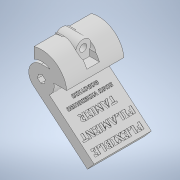
# Autodesk Inventor part: switch curvey lever boi
Saved by Autodesk Inventor 2022 (Build 260153000, 153)
## iProperties
Created: 2022-10-11
Part Number: switch curvey lever boi
Material: Generic
Document SubType Name: Modeling
Designer: Admin
Density: 1 g/cm^3
Appearance: Default
Author: Admin
Autodesk Inventor part; units mm, degrees
ref_plane "YZ Plane" through (0, 0, 0) normal (1, 0, 0) x (0, 1, 0)
ref_plane "XZ Plane" through (0, 0, 0) normal (0, 1, 0) x (-1, 0, 0)
sketch "Sketch1" plane through (0, 0, 0) normal (0, 0, 1) x (1, 0, 0)
  arc A0 (17.7715, 26.4992) -> (-7.9449, 43.6347) centre (-2.1282, 24.4992) ccw
  arc A1 (4.505, 34.4992) -> (-7.9449, 34.9952) centre (-2.1282, 24.4992) ccw
  line L0 (-2.1282, 34.4992) -> (4.505, 34.4992)
  line L1 (7.6697, 26.4992) -> (17.7715, 26.4992)
  line L2 (-8.5561, 16.8387) -> (34.0976, -18.9519)
  line L3 (34.0976, -18.9519) -> (39.2399, -12.8236)
  line L4 (39.2399, -12.8236) -> (4.0919, 16.6691)
  circle A2 centre (-2.1282, 24.4992) radius 4.5861 construction
  line L5 (-4.6095, 26.4808) -> (-1.6527, 27.6388)
  line L6 (-1.6527, 27.6388) -> (0.8285, 25.6572)
  line L7 (0.8285, 25.6572) -> (0.353, 22.5176)
  line L8 (0.353, 22.5176) -> (-2.6038, 21.3596)
  line L9 (-2.6038, 21.3596) -> (-5.085, 23.3412)
  line L10 (-5.085, 23.3412) -> (-4.6095, 26.4808)
  arc A3 (-2.1282, 34.4992) -> (-8.5561, 16.8387) centre (-2.1282, 24.4992) ccw
  arc A4 (4.0919, 16.6691) -> (7.6697, 26.4992) centre (-2.1282, 24.4992) ccw
  circle A5 centre (-2.1282, 24.4992) radius 20.0723 construction
  line L11 (-7.9449, 34.9952) -> (-7.9449, 43.7102)
  line L12 (8.708, 44.4992) -> (-7.9449, 44.4992)
  line L13 (-7.9449, 44.4992) -> (-7.9449, 31.8089)
  line L14 (-7.9449, 31.8089) -> (8.708, 31.8089)
  line L15 (8.708, 31.8089) -> (8.708, 44.4992)
  line L16 (8.708, 31.8089) -> (23.6844, 31.8089)
  line L17 (23.6844, 31.8089) -> (23.6844, 44.6206)
  line L18 (23.6844, 44.6206) -> (8.708, 44.6206)
  line L19 (8.708, 44.6206) -> (8.708, 31.8089)
  point P0 (0, 0)
  point P1 (-4.0178, 44.4097)
  point P2 (11.1125, 52.4992)
  point P3 (10.8839, 39.6875)
  point P4 (-7.9449, 34.9952)
  point P5 (8.708, 41.3092)
  point P6 (-7.9449, 32.6335)
  point P7 (-2.1282, 44.4992)
  dimension "d9" = 8
  dimension "d10" = 9.1722
  dimension "d11" = 5.5
  dimension "d12" = 40
  dimension "d13" = 8
  dimension "d16" = 8
  dimension "d17" = 10
  dimension "d18" = 20
  constraints: 40 end point, 9 point on circle, 6 parallel, 5 centre point, 4 coincident, 4 tangent, 3 perpendicular, 2 horizontal, 2 point on line, 1 vertical, 16 other
  measures "d9" distance between parallel lines of L1 L0
  measures "d10" diameter of A2
  measures "d11" distance between parallel lines of L8 L5
  measures "d12" angle of L2 L0
  measures "d13" distance between parallel lines of L2 L4
  measures "d16" radial gap between concentric circles of A0 A1
  measures "d17" radius of A3
  measures "d18" radius of A0
extrude "Extrusion1" add sketch "Sketch1" against normal blind 45 contours L1 A4 L4 L3 L2 A3 L13 L14 L16 A0 | L16 L15 A0 | L15 L14 L13 A3 L0 A1 L11 A0
ref_plane "Work Plane1" through (0, 0, -27) normal (0, 0, -1) x (-1, 0, 0)
extrude "Extrusion4" add sketch "Sketch1" along normal blind 10 from surface at -27 contours L15 L14 L13 A3 L0 A1 L11 A0 | A0 L12 L15 | A0 L11 L13 L12 | L13 A1 L0 A3
extrude "Extrusion5" cut sketch "Sketch1" along normal blind 10 from surface at -27 contours L16 L15 A0 | A0 L15 L19 L18 L17 L16 | L13 A1 L0 A3
sketch "Sketch2" plane through (8.708, 44.4992, -17) normal (1, 0, 0) x (0, 0, -1)
  circle A0 centre (5, -4.5078) radius 2.8
  line L0 (10, 0) -> (0, 0) projected
  line L1 (0, -12.6903) -> (0, -3.19) projected
  line L2 (10, 0) -> (0, 0) construction
  line L3 (5, 0) -> (5, -12.8117) construction
  circle A1 centre (5, -4.5078) radius 6
  line L4 (0, -3.19) -> (0, 0) projected
  line L5 (10, -3.19) -> (10, 0) projected
  point P0 (-17, -44.4992)
  point P1 (1.0402, 0)
  point P2 (8.9598, 0)
  point P3 (10, -1.1911)
  point P4 (0, -1.1911)
  dimension "d24" = 5.6
  dimension "d25" = 4.5078
  dimension "d29" = 12
  constraints: 2 centre point, 2 end point, 1 midpoint, 1 perpendicular, 1 point on line
  measures "d24" diameter of A0
  measures "d25" distance from line of A0.centre L0
  measures "d29" diameter of A1
extrude "Extrusion6" cut sketch "Sketch2" against normal through all contours A0
extrude "Extrusion7" cut sketch "Sketch2" along normal blind 10 contours A1 L1 L4 L0 | L0 A1 | L4 L1 A1
extrude "Extrusion8" add sketch "Sketch2" against normal up to surface (16.6529 mm away) contours A1 L1 L4 L0 | L0 A1 | L4 L1 A1
extrude "Extrusion9" cut sketch "Sketch2" against normal up to surface contours L5 A1 L0 | A1 L4 L0 round surface about axis through (-2.1282, 24.4992, 0) along (0, 0, -1) radius 20 far side no
sketch "Sketch3" plane through (39.2399, -12.8236, 0) normal (0.6427876, 0.7660444, 0) x (0.7660444, -0.6427876, 0)
  line L0 (-3.0027, 42.1524) -> (-3.0027, 2.7889) construction
  line L1 (-3.0027, 2.7889) -> (-46.5097, 2.7889) construction
  line L2 (-46.5097, 2.7889) -> (-46.5097, 42.1524) construction
  line L3 (-46.5097, 42.1524) -> (-3.0027, 42.1524) construction
  line L4 (-3.0027, 41.6774) -> (-3.0027, 40.0154)
  line L5 (-3.0027, 40.0154) -> (-5.2343, 40.0154)
  line L6 (-5.2343, 40.0154) -> (-5.2343, 38.4806)
  line L7 (-5.2343, 38.4806) -> (-6.2183, 38.4806)
  line L8 (-6.2183, 38.4806) -> (-6.2183, 40.0154)
  line L9 (-6.2183, 40.0154) -> (-8.0027, 40.0154)
  line L10 (-8.0027, 40.0154) -> (-8.0027, 41.6774)
  line L11 (-8.0027, 41.6774) -> (-3.0027, 41.6774)
  line L12 (-4.0008, 39.7517) -> (-3.0027, 39.7517)
  line L13 (-3.0027, 39.7517) -> (-3.0027, 37.2141)
  line L14 (-3.0027, 37.2141) -> (-4.6599, 37.2141)
  line L15 (-4.6599, 37.2141) -> (-4.6599, 38.876)
  line L16 (-4.6599, 38.876) -> (-4.0008, 38.876)
  line L17 (-4.0008, 38.876) -> (-4.0008, 39.7517)
  line L18 (-8.0027, 36.6726) -> (-3.0027, 36.6726)
  line L19 (-3.0027, 36.6726) -> (-3.0027, 35.0107)
  line L20 (-3.0027, 35.0107) -> (-8.0027, 35.0107)
  line L21 (-8.0027, 35.0107) -> (-8.0027, 36.6726)
  line L22 (-8.0027, 34.747) -> (-7.0046, 34.747)
  line L23 (-7.0046, 34.747) -> (-7.0046, 33.9231)
  line L24 (-7.0046, 33.9231) -> (-6.3737, 33.9231)
  line L25 (-6.3737, 33.9231) -> (-6.3737, 32.4118)
  line L26 (-6.3737, 32.4118) -> (-8.0027, 32.4118)
  line L27 (-8.0027, 32.4118) -> (-8.0027, 34.747)
  line L28 (-5.9499, 30.2367) -> (-8.0027, 30.2367)
  line L29 (-8.0027, 30.2367) -> (-8.0027, 31.8986)
  line L30 (-8.0027, 31.8986) -> (-3.0027, 31.8986)
  line L31 (-3.0027, 31.8986) -> (-3.0027, 30.2367)
  line L32 (-3.0027, 30.2367) -> (-4.9848, 30.2367)
  line L33 (-4.9848, 30.2367) -> (-4.9848, 28.6453)
  line L34 (-4.9848, 28.6453) -> (-5.9499, 28.6453)
  line L35 (-5.9499, 28.6453) -> (-5.9499, 30.2367)
  line L36 (-8.0027, 29.973) -> (-7.0046, 29.973)
  line L37 (-7.0046, 29.973) -> (-7.0046, 29.0361)
  line L38 (-7.0046, 29.0361) -> (-6.5055, 29.0361)
  line L39 (-6.5055, 29.0361) -> (-6.5055, 27.3694)
  line L40 (-6.5055, 27.3694) -> (-8.0027, 27.3694)
  line L41 (-8.0027, 27.3694) -> (-8.0027, 29.973)
  line L42 (-3.9725, 29.973) -> (-3.0027, 29.973)
  line L43 (-3.0027, 29.973) -> (-3.0027, 27.3694)
  line L44 (-3.0027, 27.3694) -> (-4.4528, 27.3694)
  line L45 (-4.4528, 27.3694) -> (-4.4528, 28.9372)
  line L46 (-4.4528, 28.9372) -> (-3.9725, 28.9372)
  line L47 (-3.9725, 28.9372) -> (-3.9725, 29.973)
  line L48 (-8.0027, 21.861) -> (-8.0027, 23.6736)
  line L49 (-8.0027, 23.6736) -> (-3.0027, 27.0069)
  line L50 (-3.0027, 27.0069) -> (-3.0027, 25.2131)
  line L51 (-3.0027, 25.2131) -> (-8.0027, 21.861)
  line L52 (-8.0027, 27.1105) -> (-5.7098, 25.5145)
  line L53 (-5.7098, 25.5145) -> (-7.0469, 24.6246)
  line L54 (-7.0469, 24.6246) -> (-8.0027, 25.2084)
  line L55 (-8.0027, 25.2084) -> (-8.0027, 27.1105)
  line L56 (-5.3049, 23.4099) -> (-4.0243, 24.2998)
  line L57 (-4.0243, 24.2998) -> (-3.0027, 23.716)
  line L58 (-3.0027, 23.716) -> (-3.0027, 21.9316)
  line L59 (-3.0027, 21.9316) -> (-5.3049, 23.4099)
  line L60 (-6.9339, 21.5879) -> (-6.9339, 21.0888)
  line L61 (-6.9339, 21.0888) -> (-4.0667, 21.0888)
  line L62 (-4.0667, 21.0888) -> (-4.0667, 21.5879)
  line L63 (-4.0667, 21.5879) -> (-3.0027, 21.5879)
  line L64 (-3.0027, 21.5879) -> (-3.0027, 18.9231)
  line L65 (-3.0027, 18.9231) -> (-4.0667, 18.9231)
  line L66 (-4.0667, 18.9231) -> (-4.0667, 19.4269)
  line L67 (-4.0667, 19.4269) -> (-6.9339, 19.4269)
  line L68 (-6.9339, 19.4269) -> (-6.9339, 18.9231)
  line L69 (-6.9339, 18.9231) -> (-8.0027, 18.9231)
  line L70 (-8.0027, 18.9231) -> (-8.0027, 21.5879)
  line L71 (-8.0027, 21.5879) -> (-6.9339, 21.5879)
  line L72 (-4.0008, 14.9542) -> (-4.0008, 16.1877)
  line L73 (-4.0008, 16.1877) -> (-3.0027, 16.1877)
  line L74 (-3.0027, 16.1877) -> (-3.0027, 14.2574)
  line L75 (-3.0027, 14.2574) -> (-4.0008, 13.2546)
  line L76 (-4.0008, 13.2546) -> (-5.0177, 13.2546)
  line L77 (-5.0177, 13.2546) -> (-5.5168, 13.7536)
  line L78 (-5.5168, 13.7536) -> (-6.0206, 13.2546)
  line L79 (-6.0206, 13.2546) -> (-7.0046, 13.2546)
  line L80 (-7.0046, 13.2546) -> (-8.0027, 14.2574)
  line L81 (-8.0027, 14.2574) -> (-8.0027, 16.1877)
  line L82 (-8.0027, 16.1877) -> (-7.0046, 16.1877)
  line L83 (-7.0046, 16.1877) -> (-7.0046, 14.9542)
  line L84 (-7.0046, 14.9542) -> (-5.9358, 14.9542)
  line L85 (-5.9358, 14.9542) -> (-5.9358, 16.1877)
  line L86 (-5.9358, 16.1877) -> (-5.0648, 16.1877)
  line L87 (-5.0648, 16.1877) -> (-5.0648, 14.9542)
  line L88 (-5.0648, 14.9542) -> (-4.0008, 14.9542)
  line L89 (-3.0027, 18.1133) -> (-3.0027, 16.4514)
  line L90 (-3.0027, 16.4514) -> (-8.0027, 16.4514)
  line L91 (-8.0027, 16.4514) -> (-8.0027, 18.1133)
  line L92 (-8.0027, 18.1133) -> (-3.0027, 18.1133)
  line L93 (-8.0027, 12.4824) -> (-3.0027, 12.4824)
  line L94 (-3.0027, 12.4824) -> (-3.0027, 10.8205)
  line L95 (-3.0027, 10.8205) -> (-8.0027, 10.8205)
  line L96 (-8.0027, 10.8205) -> (-8.0027, 12.4824)
  line L97 (-8.0027, 10.5568) -> (-7.0046, 10.5568)
  line L98 (-7.0046, 10.5568) -> (-7.0046, 9.7329)
  line L99 (-7.0046, 9.7329) -> (-6.3737, 9.7329)
  line L100 (-6.3737, 9.7329) -> (-6.3737, 8.2216)
  line L101 (-6.3737, 8.2216) -> (-8.0027, 8.2216)
  line L102 (-8.0027, 8.2216) -> (-8.0027, 10.5568)
  line L103 (-5.9499, 6.0465) -> (-8.0027, 6.0465)
  line L104 (-8.0027, 6.0465) -> (-8.0027, 7.7084)
  line L105 (-8.0027, 7.7084) -> (-3.0027, 7.7084)
  line L106 (-3.0027, 7.7084) -> (-3.0027, 6.0465)
  line L107 (-3.0027, 6.0465) -> (-4.9848, 6.0465)
  line L108 (-4.9848, 6.0465) -> (-4.9848, 4.4551)
  line L109 (-4.9848, 4.4551) -> (-5.9499, 4.4551)
  line L110 (-5.9499, 4.4551) -> (-5.9499, 6.0465)
  line L111 (-8.0027, 5.7828) -> (-7.0046, 5.7828)
  line L112 (-7.0046, 5.7828) -> (-7.0046, 4.8459)
  line L113 (-7.0046, 4.8459) -> (-6.5055, 4.8459)
  line L114 (-6.5055, 4.8459) -> (-6.5055, 3.1792)
  line L115 (-6.5055, 3.1792) -> (-8.0027, 3.1792)
  line L116 (-8.0027, 3.1792) -> (-8.0027, 5.7828)
  line L117 (-3.9725, 5.7828) -> (-3.0027, 5.7828)
  line L118 (-3.0027, 5.7828) -> (-3.0027, 3.1792)
  line L119 (-3.0027, 3.1792) -> (-4.4528, 3.1792)
  line L120 (-4.4528, 3.1792) -> (-4.4528, 4.747)
  line L121 (-4.4528, 4.747) -> (-3.9725, 4.747)
  line L122 (-3.9725, 4.747) -> (-3.9725, 5.7828)
  line L123 (-13.1117, 42.7908) -> (-13.1117, 41.1289)
  line L124 (-13.1117, 41.1289) -> (-15.3433, 41.1289)
  line L125 (-15.3433, 41.1289) -> (-15.3433, 39.594)
  line L126 (-15.3433, 39.594) -> (-16.3273, 39.594)
  line L127 (-16.3273, 39.594) -> (-16.3273, 41.1289)
  line L128 (-16.3273, 41.1289) -> (-18.1117, 41.1289)
  line L129 (-18.1117, 41.1289) -> (-18.1117, 42.7908)
  line L130 (-18.1117, 42.7908) -> (-13.1117, 42.7908)
  line L131 (-14.1098, 40.8652) -> (-13.1117, 40.8652)
  line L132 (-13.1117, 40.8652) -> (-13.1117, 38.3275)
  line L133 (-13.1117, 38.3275) -> (-14.7689, 38.3275)
  line L134 (-14.7689, 38.3275) -> (-14.7689, 39.9895)
  line L135 (-14.7689, 39.9895) -> (-14.1098, 39.9895)
  line L136 (-14.1098, 39.9895) -> (-14.1098, 40.8652)
  line L137 (-17.043, 37.8614) -> (-17.043, 37.3624)
  line L138 (-17.043, 37.3624) -> (-14.1757, 37.3624)
  line L139 (-14.1757, 37.3624) -> (-14.1757, 37.8614)
  line L140 (-14.1757, 37.8614) -> (-13.1117, 37.8614)
  line L141 (-13.1117, 37.8614) -> (-13.1117, 35.1967)
  line L142 (-13.1117, 35.1967) -> (-14.1757, 35.1967)
  line L143 (-14.1757, 35.1967) -> (-14.1757, 35.7004)
  line L144 (-14.1757, 35.7004) -> (-17.043, 35.7004)
  line L145 (-17.043, 35.7004) -> (-17.043, 35.1967)
  line L146 (-17.043, 35.1967) -> (-18.1117, 35.1967)
  line L147 (-18.1117, 35.1967) -> (-18.1117, 37.8614)
  line L148 (-18.1117, 37.8614) -> (-17.043, 37.8614)
  line L149 (-18.1117, 34.3869) -> (-13.1117, 34.3869)
  line L150 (-13.1117, 34.3869) -> (-13.1117, 32.7249)
  line L151 (-13.1117, 32.7249) -> (-18.1117, 32.7249)
  line L152 (-18.1117, 32.7249) -> (-18.1117, 34.3869)
  line L153 (-18.1117, 32.4612) -> (-17.1136, 32.4612)
  line L154 (-17.1136, 32.4612) -> (-17.1136, 31.6373)
  line L155 (-17.1136, 31.6373) -> (-16.4827, 31.6373)
  line L156 (-16.4827, 31.6373) -> (-16.4827, 30.126)
  line L157 (-16.4827, 30.126) -> (-18.1117, 30.126)
  line L158 (-18.1117, 30.126) -> (-18.1117, 32.4612)
  line L159 (-17.5656, 26.336) -> (-17.5656, 27.9697)
  line L160 (-17.5656, 27.9697) -> (-16.5721, 27.6213)
  line L161 (-16.5721, 27.6213) -> (-16.5721, 26.7174)
  line L162 (-16.5721, 26.7174) -> (-13.1117, 28.0545)
  line L163 (-13.1117, 28.0545) -> (-13.1117, 26.4349)
  line L164 (-13.1117, 26.4349) -> (-18.1117, 24.4386)
  line L165 (-18.1117, 24.4386) -> (-18.1117, 26.1241)
  line L166 (-18.1117, 26.1241) -> (-17.5656, 26.336)
  line L167 (-18.1117, 28.4123) -> (-18.1117, 30.0225)
  line L168 (-18.1117, 30.0225) -> (-13.3848, 28.2381)
  line L169 (-13.3848, 28.2381) -> (-15.3386, 27.4989)
  line L170 (-15.3386, 27.4989) -> (-18.1117, 28.4123)
  line L171 (-13.1117, 23.9631) -> (-13.1117, 22.1929)
  line L172 (-13.1117, 22.1929) -> (-15.3763, 20.8511)
  line L173 (-15.3763, 20.8511) -> (-13.5966, 19.7965)
  line L174 (-13.5966, 19.7965) -> (-16.0731, 19.7965)
  line L175 (-16.0731, 19.7965) -> (-18.1117, 20.997)
  line L176 (-18.1117, 20.997) -> (-13.1117, 23.9631)
  line L177 (-18.1117, 19.5516) -> (-13.1117, 19.5516)
  line L178 (-13.1117, 19.5516) -> (-13.1117, 17.8897)
  line L179 (-13.1117, 17.8897) -> (-18.1117, 17.8897)
  line L180 (-18.1117, 17.8897) -> (-18.1117, 19.5516)
  line L181 (-18.1117, 23.9631) -> (-13.6437, 23.9631)
  line L182 (-13.6437, 23.9631) -> (-16.2143, 22.4095)
  line L183 (-16.2143, 22.4095) -> (-18.1117, 22.4095)
  line L184 (-18.1117, 22.4095) -> (-18.1117, 23.9631)
  line L185 (-16.059, 15.3426) -> (-18.1117, 15.3426)
  line L186 (-18.1117, 15.3426) -> (-18.1117, 17.0046)
  line L187 (-18.1117, 17.0046) -> (-13.1117, 17.0046)
  line L188 (-13.1117, 17.0046) -> (-13.1117, 15.3426)
  line L189 (-13.1117, 15.3426) -> (-15.0938, 15.3426)
  line L190 (-15.0938, 15.3426) -> (-15.0938, 13.7513)
  line L191 (-15.0938, 13.7513) -> (-16.059, 13.7513)
  line L192 (-16.059, 13.7513) -> (-16.059, 15.3426)
  line L193 (-18.1117, 15.079) -> (-17.1136, 15.079)
  line L194 (-17.1136, 15.079) -> (-17.1136, 14.142)
  line L195 (-17.1136, 14.142) -> (-16.6145, 14.142)
  line L196 (-16.6145, 14.142) -> (-16.6145, 12.4754)
  line L197 (-16.6145, 12.4754) -> (-18.1117, 12.4754)
  line L198 (-18.1117, 12.4754) -> (-18.1117, 15.079)
  line L199 (-14.0816, 15.079) -> (-13.1117, 15.079)
  line L200 (-13.1117, 15.079) -> (-13.1117, 12.4754)
  line L201 (-13.1117, 12.4754) -> (-14.5618, 12.4754)
  line L202 (-14.5618, 12.4754) -> (-14.5618, 14.0432)
  line L203 (-14.5618, 14.0432) -> (-14.0816, 14.0432)
  line L204 (-14.0816, 14.0432) -> (-14.0816, 15.079)
  line L205 (-18.1117, 6.8774) -> (-18.1117, 8.6477)
  line L206 (-18.1117, 8.6477) -> (-13.1117, 11.675)
  line L207 (-13.1117, 11.675) -> (-13.1117, 9.9189)
  line L208 (-13.1117, 9.9189) -> (-18.1117, 6.8774)
  line L209 (-13.1117, 6.8774) -> (-17.6456, 6.8774)
  line L210 (-17.6456, 6.8774) -> (-15.2915, 8.3275)
  line L211 (-15.2915, 8.3275) -> (-13.1117, 8.3275)
  line L212 (-13.1117, 8.3275) -> (-13.1117, 6.8774)
  line L213 (-18.1117, 11.675) -> (-13.6578, 11.675)
  line L214 (-13.6578, 11.675) -> (-15.9978, 10.2249)
  line L215 (-15.9978, 10.2249) -> (-18.1117, 10.2249)
  line L216 (-18.1117, 10.2249) -> (-18.1117, 11.675)
  line L217 (-14.4582, 4.9424) -> (-14.4582, 3.2098)
  line L218 (-14.4582, 3.2098) -> (-18.1117, 3.2098)
  line L219 (-18.1117, 3.2098) -> (-18.1117, 4.9424)
  line L220 (-18.1117, 4.9424) -> (-14.4582, 4.9424)
  line L221 (-13.1117, 6.2419) -> (-13.1117, 1.9057)
  line L222 (-13.1117, 1.9057) -> (-14.1993, 1.9057)
  line L223 (-14.1993, 1.9057) -> (-14.1993, 6.2419)
  line L224 (-14.1993, 6.2419) -> (-13.1117, 6.2419)
  line L225 (-24.5672, 35.1072) -> (-24.5672, 33.3746)
  line L226 (-24.5672, 33.3746) -> (-28.2207, 33.3746)
  line L227 (-28.2207, 33.3746) -> (-28.2207, 35.1072)
  line L228 (-28.2207, 35.1072) -> (-24.5672, 35.1072)
  line L229 (-23.2207, 36.4066) -> (-23.2207, 32.0705)
  line L230 (-23.2207, 32.0705) -> (-24.3083, 32.0705)
  line L231 (-24.3083, 32.0705) -> (-24.3083, 36.4066)
  line L232 (-24.3083, 36.4066) -> (-23.2207, 36.4066)
  line L233 (-27.6746, 28.1533) -> (-27.6746, 29.787)
  line L234 (-27.6746, 29.787) -> (-26.6812, 29.4387)
  line L235 (-26.6812, 29.4387) -> (-26.6812, 28.5347)
  line L236 (-26.6812, 28.5347) -> (-23.2207, 29.8718)
  line L237 (-23.2207, 29.8718) -> (-23.2207, 28.2522)
  line L238 (-23.2207, 28.2522) -> (-28.2207, 26.256)
  line L239 (-28.2207, 26.256) -> (-28.2207, 27.9415)
  line L240 (-28.2207, 27.9415) -> (-27.6746, 28.1533)
  line L241 (-28.2207, 30.2296) -> (-28.2207, 31.8398)
  line L242 (-28.2207, 31.8398) -> (-23.4938, 30.0554)
  line L243 (-23.4938, 30.0554) -> (-25.4476, 29.3162)
  line L244 (-25.4476, 29.3162) -> (-28.2207, 30.2296)
  line L245 (-23.2207, 25.7805) -> (-23.2207, 24.0102)
  line L246 (-23.2207, 24.0102) -> (-25.4853, 22.6684)
  line L247 (-25.4853, 22.6684) -> (-23.7056, 21.6138)
  line L248 (-23.7056, 21.6138) -> (-26.1821, 21.6138)
  line L249 (-26.1821, 21.6138) -> (-28.2207, 22.8144)
  line L250 (-28.2207, 22.8144) -> (-23.2207, 25.7805)
  line L251 (-28.2207, 21.369) -> (-23.2207, 21.369)
  line L252 (-23.2207, 21.369) -> (-23.2207, 19.707)
  line L253 (-23.2207, 19.707) -> (-28.2207, 19.707)
  line L254 (-28.2207, 19.707) -> (-28.2207, 21.369)
  line L255 (-28.2207, 25.7805) -> (-23.7527, 25.7805)
  line L256 (-23.7527, 25.7805) -> (-26.3233, 24.2268)
  line L257 (-26.3233, 24.2268) -> (-28.2207, 24.2268)
  line L258 (-28.2207, 24.2268) -> (-28.2207, 25.7805)
  line L259 (-26.168, 17.1599) -> (-28.2207, 17.1599)
  line L260 (-28.2207, 17.1599) -> (-28.2207, 18.8219)
  line L261 (-28.2207, 18.8219) -> (-23.2207, 18.8219)
  line L262 (-23.2207, 18.8219) -> (-23.2207, 17.1599)
  line L263 (-23.2207, 17.1599) -> (-25.2028, 17.1599)
  line L264 (-25.2028, 17.1599) -> (-25.2028, 15.5686)
  line L265 (-25.2028, 15.5686) -> (-26.168, 15.5686)
  line L266 (-26.168, 15.5686) -> (-26.168, 17.1599)
  line L267 (-28.2207, 16.8963) -> (-27.2226, 16.8963)
  line L268 (-27.2226, 16.8963) -> (-27.2226, 15.9594)
  line L269 (-27.2226, 15.9594) -> (-26.7235, 15.9594)
  line L270 (-26.7235, 15.9594) -> (-26.7235, 14.2927)
  line L271 (-26.7235, 14.2927) -> (-28.2207, 14.2927)
  line L272 (-28.2207, 14.2927) -> (-28.2207, 16.8963)
  line L273 (-24.1906, 16.8963) -> (-23.2207, 16.8963)
  line L274 (-23.2207, 16.8963) -> (-23.2207, 14.2927)
  line L275 (-23.2207, 14.2927) -> (-24.6708, 14.2927)
  line L276 (-24.6708, 14.2927) -> (-24.6708, 15.8605)
  line L277 (-24.6708, 15.8605) -> (-24.1906, 15.8605)
  line L278 (-24.1906, 15.8605) -> (-24.1906, 16.8963)
  line L279 (-28.2207, 13.4923) -> (-23.2207, 13.4923)
  line L280 (-23.2207, 13.4923) -> (-23.2207, 11.8304)
  line L281 (-23.2207, 11.8304) -> (-28.2207, 11.8304)
  line L282 (-28.2207, 11.8304) -> (-28.2207, 13.4923)
  line L283 (-24.2188, 11.5667) -> (-23.2207, 11.5667)
  line L284 (-23.2207, 11.5667) -> (-23.2207, 9.6646)
  line L285 (-23.2207, 9.6646) -> (-24.2188, 8.6618)
  line L286 (-24.2188, 8.6618) -> (-25.7207, 8.6618)
  line L287 (-25.7207, 8.6618) -> (-26.4881, 9.4292)
  line L288 (-26.4881, 9.4292) -> (-26.3845, 9.4857)
  line L289 (-26.3845, 9.4857) -> (-26.587, 11.0488)
  line L290 (-26.587, 11.0488) -> (-26.7188, 10.9876)
  line L291 (-26.7188, 10.9876) -> (-26.7188, 11.5667)
  line L292 (-26.7188, 11.5667) -> (-25.7537, 11.5667)
  line L293 (-25.7537, 11.5667) -> (-25.7537, 10.3144)
  line L294 (-25.7537, 10.3144) -> (-24.2188, 10.3144)
  line L295 (-24.2188, 10.3144) -> (-24.2188, 11.5667)
  line L296 (-28.2207, 8.4923) -> (-28.2207, 10.272)
  line L297 (-28.2207, 10.272) -> (-26.7188, 10.9876)
  line L298 (-26.7188, 10.9876) -> (-26.7188, 9.6646)
  line L299 (-26.7188, 9.6646) -> (-26.4881, 9.4292)
  line L300 (-26.4881, 9.4292) -> (-28.2207, 8.4923)
  line L301 (-34.8868, 39.3104) -> (-34.8868, 40.1437)
  line L302 (-34.8868, 40.1437) -> (-33.9899, 40.1437)
  line L303 (-33.9899, 40.1437) -> (-33.4885, 39.6093)
  line L304 (-33.4885, 39.6093) -> (-33.4885, 38.6253)
  line L305 (-33.4885, 38.6253) -> (-32.3868, 38.6253)
  line L306 (-32.3868, 38.6253) -> (-32.3868, 38.2911)
  line L307 (-32.3868, 38.2911) -> (-32.8858, 37.792)
  line L308 (-32.8858, 37.792) -> (-33.5049, 37.792)
  line L309 (-33.5049, 37.792) -> (-34.004, 38.2911)
  line L310 (-34.004, 38.2911) -> (-34.004, 39.3104)
  line L311 (-34.004, 39.3104) -> (-34.8868, 39.3104)
  line L312 (-32.8364, 39.3104) -> (-33.2013, 39.3104)
  line L313 (-33.2013, 39.3104) -> (-33.2013, 40.1437)
  line L314 (-33.2013, 40.1437) -> (-32.8858, 40.1437)
  line L315 (-32.8858, 40.1437) -> (-32.3868, 39.6423)
  line L316 (-32.3868, 39.6423) -> (-32.3868, 38.7572)
  line L317 (-32.3868, 38.7572) -> (-32.8364, 38.7572)
  line L318 (-32.8364, 38.7572) -> (-32.8364, 39.3104)
  line L319 (-34.8868, 39.1785) -> (-34.4371, 39.1785)
  line L320 (-34.4371, 39.1785) -> (-34.4371, 37.792)
  line L321 (-34.4371, 37.792) -> (-34.8868, 37.792)
  line L322 (-34.8868, 37.792) -> (-34.8868, 39.1785)
  line L323 (-34.3877, 34.9695) -> (-34.8868, 35.4685)
  line L324 (-34.8868, 35.4685) -> (-34.8868, 36.4266)
  line L325 (-34.8868, 36.4266) -> (-34.3877, 36.4266)
  line L326 (-34.3877, 36.4266) -> (-34.3877, 35.8028)
  line L327 (-34.3877, 35.8028) -> (-32.3868, 35.8028)
  line L328 (-32.3868, 35.8028) -> (-32.3868, 35.4685)
  line L329 (-32.3868, 35.4685) -> (-32.8858, 34.9695)
  line L330 (-32.8858, 34.9695) -> (-34.3877, 34.9695)
  line L331 (-34.8868, 36.5538) -> (-34.8868, 36.8857)
  line L332 (-34.8868, 36.8857) -> (-34.3877, 37.3871)
  line L333 (-34.3877, 37.3871) -> (-32.8858, 37.3871)
  line L334 (-32.8858, 37.3871) -> (-32.3868, 36.8857)
  line L335 (-32.3868, 36.8857) -> (-32.3868, 35.9299)
  line L336 (-32.3868, 35.9299) -> (-32.8858, 35.9299)
  line L337 (-32.8858, 35.9299) -> (-32.8858, 36.5538)
  line L338 (-32.8858, 36.5538) -> (-34.8868, 36.5538)
  line L339 (-34.8868, 33.7313) -> (-34.8868, 34.5646)
  line L340 (-34.8868, 34.5646) -> (-33.9899, 34.5646)
  line L341 (-33.9899, 34.5646) -> (-33.4885, 34.0302)
  line L342 (-33.4885, 34.0302) -> (-33.4885, 33.0462)
  line L343 (-33.4885, 33.0462) -> (-32.3868, 33.0462)
  line L344 (-32.3868, 33.0462) -> (-32.3868, 32.712)
  line L345 (-32.3868, 32.712) -> (-32.8858, 32.2129)
  line L346 (-32.8858, 32.2129) -> (-33.5049, 32.2129)
  line L347 (-33.5049, 32.2129) -> (-34.004, 32.712)
  line L348 (-34.004, 32.712) -> (-34.004, 33.7313)
  line L349 (-34.004, 33.7313) -> (-34.8868, 33.7313)
  line L350 (-32.8364, 33.7313) -> (-33.2013, 33.7313)
  line L351 (-33.2013, 33.7313) -> (-33.2013, 34.5646)
  line L352 (-33.2013, 34.5646) -> (-32.8858, 34.5646)
  line L353 (-32.8858, 34.5646) -> (-32.3868, 34.0632)
  line L354 (-32.3868, 34.0632) -> (-32.3868, 33.1781)
  line L355 (-32.3868, 33.1781) -> (-32.8364, 33.1781)
  line L356 (-32.8364, 33.1781) -> (-32.8364, 33.7313)
  line L357 (-34.8868, 33.5994) -> (-34.4371, 33.5994)
  line L358 (-34.4371, 33.5994) -> (-34.4371, 32.2129)
  line L359 (-34.4371, 32.2129) -> (-34.8868, 32.2129)
  line L360 (-34.8868, 32.2129) -> (-34.8868, 33.5994)
  line L361 (-32.3868, 29.8989) -> (-32.8858, 29.3998)
  line L362 (-32.8858, 29.3998) -> (-33.3778, 29.3998)
  line L363 (-33.3778, 29.3998) -> (-33.6297, 29.6941)
  line L364 (-33.6297, 29.6941) -> (-33.8839, 29.3998)
  line L365 (-33.8839, 29.3998) -> (-34.3901, 29.3998)
  line L366 (-34.3901, 29.3998) -> (-34.8868, 29.8989)
  line L367 (-34.8868, 29.8989) -> (-34.8868, 30.2331)
  line L368 (-34.8868, 30.2331) -> (-33.8321, 30.2331)
  line L369 (-33.8321, 30.2331) -> (-33.8321, 30.8122)
  line L370 (-33.8321, 30.8122) -> (-33.3966, 30.8122)
  line L371 (-33.3966, 30.8122) -> (-33.3966, 30.2331)
  line L372 (-33.3966, 30.2331) -> (-32.3868, 30.2331)
  line L373 (-32.3868, 30.2331) -> (-32.3868, 29.8989)
  line L374 (-32.9188, 30.9817) -> (-33.2837, 30.9817)
  line L375 (-33.2837, 30.9817) -> (-33.2837, 31.8151)
  line L376 (-33.2837, 31.8151) -> (-32.8858, 31.8151)
  line L377 (-32.8858, 31.8151) -> (-32.3868, 31.316)
  line L378 (-32.3868, 31.316) -> (-32.3868, 30.365)
  line L379 (-32.3868, 30.365) -> (-32.9188, 30.365)
  line L380 (-32.9188, 30.365) -> (-32.9188, 30.9817)
  line L381 (-34.3877, 31.8151) -> (-34.0016, 31.8151)
  line L382 (-34.0016, 31.8151) -> (-34.0016, 30.9817)
  line L383 (-34.0016, 30.9817) -> (-34.3524, 30.9817)
  line L384 (-34.3524, 30.9817) -> (-34.3524, 30.365)
  line L385 (-34.3524, 30.365) -> (-34.8868, 30.365)
  line L386 (-34.8868, 30.365) -> (-34.8868, 31.316)
  line L387 (-34.8868, 31.316) -> (-34.3877, 31.8151)
  line L388 (-34.8868, 26.5326) -> (-34.8868, 27.3424)
  line L389 (-34.8868, 27.3424) -> (-32.3868, 28.2463)
  line L390 (-32.3868, 28.2463) -> (-32.3868, 27.3965)
  line L391 (-32.3868, 27.3965) -> (-34.8868, 26.5326)
  line L392 (-32.3868, 26.4031) -> (-32.3868, 25.5674)
  line L393 (-32.3868, 25.5674) -> (-34.8114, 26.4314)
  line L394 (-34.8114, 26.4314) -> (-33.7286, 26.8056)
  line L395 (-33.7286, 26.8056) -> (-32.3868, 26.4031)
  line L396 (-34.3524, 25.4309) -> (-34.3524, 25.1814)
  line L397 (-34.3524, 25.1814) -> (-32.9188, 25.1814)
  line L398 (-32.9188, 25.1814) -> (-32.9188, 25.4309)
  line L399 (-32.9188, 25.4309) -> (-32.3868, 25.4309)
  line L400 (-32.3868, 25.4309) -> (-32.3868, 24.0985)
  line L401 (-32.3868, 24.0985) -> (-32.9188, 24.0985)
  line L402 (-32.9188, 24.0985) -> (-32.9188, 24.3504)
  line L403 (-32.9188, 24.3504) -> (-34.3524, 24.3504)
  line L404 (-34.3524, 24.3504) -> (-34.3524, 24.0985)
  line L405 (-34.3524, 24.0985) -> (-34.8868, 24.0985)
  line L406 (-34.8868, 24.0985) -> (-34.8868, 25.4309)
  line L407 (-34.8868, 25.4309) -> (-34.3524, 25.4309)
  line L408 (-34.8868, 22.9003) -> (-34.8868, 23.2322)
  line L409 (-34.8868, 23.2322) -> (-34.3877, 23.7313)
  line L410 (-34.3877, 23.7313) -> (-32.8858, 23.7313)
  line L411 (-32.8858, 23.7313) -> (-32.3868, 23.2322)
  line L412 (-32.3868, 23.2322) -> (-32.3868, 22.9003)
  line L413 (-32.3868, 22.9003) -> (-34.8868, 22.9003)
  line L414 (-32.8858, 22.7685) -> (-32.3868, 22.7685)
  line L415 (-32.3868, 22.7685) -> (-32.3868, 21.881)
  line L416 (-32.3868, 21.881) -> (-32.8858, 21.3819)
  line L417 (-32.8858, 21.3819) -> (-33.3896, 21.3819)
  line L418 (-33.3896, 21.3819) -> (-33.3896, 22.2153)
  line L419 (-33.3896, 22.2153) -> (-32.8858, 22.2153)
  line L420 (-32.8858, 22.2153) -> (-32.8858, 22.7685)
  line L421 (-34.8868, 22.7685) -> (-34.3877, 22.7685)
  line L422 (-34.3877, 22.7685) -> (-34.3877, 22.2153)
  line L423 (-34.3877, 22.2153) -> (-34.0228, 22.2153)
  line L424 (-34.0228, 22.2153) -> (-34.0228, 21.3819)
  line L425 (-34.0228, 21.3819) -> (-34.3877, 21.3819)
  line L426 (-34.3877, 21.3819) -> (-34.8868, 21.881)
  line L427 (-34.8868, 21.881) -> (-34.8868, 22.7685)
  line L428 (-34.8868, 20.9817) -> (-32.3868, 20.9817)
  line L429 (-32.3868, 20.9817) -> (-32.3868, 20.1507)
  line L430 (-32.3868, 20.1507) -> (-34.8868, 20.1507)
  line L431 (-34.8868, 20.1507) -> (-34.8868, 20.9817)
  line L432 (-34.5384, 20.0236) -> (-33.3425, 20.0236)
  line L433 (-33.3425, 20.0236) -> (-32.3868, 19.4398)
  line L434 (-32.3868, 19.4398) -> (-32.3868, 18.5735)
  line L435 (-32.3868, 18.5735) -> (-34.5384, 20.0236)
  line L436 (-34.8868, 18.5335) -> (-34.8868, 19.4328)
  line L437 (-34.8868, 19.4328) -> (-34.3147, 19.7153)
  line L438 (-34.3147, 19.7153) -> (-33.585, 19.2233)
  line L439 (-33.585, 19.2233) -> (-34.8868, 18.5335)
  line L440 (-34.8868, 16.8598) -> (-33.9498, 16.8598)
  line L441 (-33.9498, 16.8598) -> (-33.9498, 17.9403)
  line L442 (-33.9498, 17.9403) -> (-33.4555, 18.4394)
  line L443 (-33.4555, 18.4394) -> (-32.8858, 18.4394)
  line L444 (-32.8858, 18.4394) -> (-32.3868, 17.9403)
  line L445 (-32.3868, 17.9403) -> (-32.3868, 17.6578)
  line L446 (-32.3868, 17.6578) -> (-33.2742, 17.6578)
  line L447 (-33.2742, 17.6578) -> (-33.2742, 16.509)
  line L448 (-33.2742, 16.509) -> (-33.778, 16.0241)
  line L449 (-33.778, 16.0241) -> (-34.3877, 16.0241)
  line L450 (-34.3877, 16.0241) -> (-34.8868, 16.5232)
  line L451 (-34.8868, 16.5232) -> (-34.8868, 16.8598)
  line L452 (-34.1358, 18.4394) -> (-34.1358, 17.6084)
  line L453 (-34.1358, 17.6084) -> (-34.4348, 17.6084)
  line L454 (-34.4348, 17.6084) -> (-34.4348, 16.9916)
  line L455 (-34.4348, 16.9916) -> (-34.8868, 16.9916)
  line L456 (-34.8868, 16.9916) -> (-34.8868, 18.0203)
  line L457 (-34.8868, 18.0203) -> (-34.3877, 18.4394)
  line L458 (-34.3877, 18.4394) -> (-34.1358, 18.4394)
  line L459 (-32.8364, 17.526) -> (-32.3868, 17.526)
  line L460 (-32.3868, 17.526) -> (-32.3868, 16.5255)
  line L461 (-32.3868, 16.5255) -> (-32.8223, 16.0924)
  line L462 (-32.8223, 16.0924) -> (-33.0859, 16.0924)
  line L463 (-33.0859, 16.0924) -> (-33.0859, 16.8598)
  line L464 (-33.0859, 16.8598) -> (-32.8364, 16.8598)
  line L465 (-32.8364, 16.8598) -> (-32.8364, 17.526)
  line L466 (-32.8858, 14.0396) -> (-32.8858, 14.6564)
  line L467 (-32.8858, 14.6564) -> (-32.3868, 14.6564)
  line L468 (-32.3868, 14.6564) -> (-32.3868, 13.6912)
  line L469 (-32.3868, 13.6912) -> (-32.8858, 13.1898)
  line L470 (-32.8858, 13.1898) -> (-33.3943, 13.1898)
  line L471 (-33.3943, 13.1898) -> (-33.6438, 13.4394)
  line L472 (-33.6438, 13.4394) -> (-33.8957, 13.1898)
  line L473 (-33.8957, 13.1898) -> (-34.3877, 13.1898)
  line L474 (-34.3877, 13.1898) -> (-34.8868, 13.6912)
  line L475 (-34.8868, 13.6912) -> (-34.8868, 14.6564)
  line L476 (-34.8868, 14.6564) -> (-34.3877, 14.6564)
  line L477 (-34.3877, 14.6564) -> (-34.3877, 14.0396)
  line L478 (-34.3877, 14.0396) -> (-33.8533, 14.0396)
  line L479 (-33.8533, 14.0396) -> (-33.8533, 14.6564)
  line L480 (-33.8533, 14.6564) -> (-33.4178, 14.6564)
  line L481 (-33.4178, 14.6564) -> (-33.4178, 14.0396)
  line L482 (-33.4178, 14.0396) -> (-32.8858, 14.0396)
  line L483 (-32.3868, 15.6192) -> (-32.3868, 14.7882)
  line L484 (-32.3868, 14.7882) -> (-34.8868, 14.7882)
  line L485 (-34.8868, 14.7882) -> (-34.8868, 15.6192)
  line L486 (-34.8868, 15.6192) -> (-32.3868, 15.6192)
  line L487 (-34.3877, 11.9916) -> (-34.3877, 11.6856)
  line L488 (-34.3877, 11.6856) -> (-34.8868, 11.6856)
  line L489 (-34.8868, 11.6856) -> (-34.8868, 12.3235)
  line L490 (-34.8868, 12.3235) -> (-34.3877, 12.8249)
  line L491 (-34.3877, 12.8249) -> (-32.3868, 12.8249)
  line L492 (-32.3868, 12.8249) -> (-32.3868, 11.9916)
  line L493 (-32.3868, 11.9916) -> (-34.3877, 11.9916)
  line L494 (-34.3877, 10.412) -> (-34.8868, 10.9111)
  line L495 (-34.8868, 10.9111) -> (-34.8868, 11.5538)
  line L496 (-34.8868, 11.5538) -> (-34.3877, 11.5538)
  line L497 (-34.3877, 11.5538) -> (-34.3877, 11.243)
  line L498 (-34.3877, 11.243) -> (-32.3868, 11.243)
  line L499 (-32.3868, 11.243) -> (-32.3868, 10.412)
  line L500 (-32.3868, 10.412) -> (-34.3877, 10.412)
  line L501 (-34.8868, 9.9883) -> (-32.3868, 9.9883)
  line L502 (-32.3868, 9.9883) -> (-32.3868, 9.1573)
  line L503 (-32.3868, 9.1573) -> (-34.8868, 9.1573)
  line L504 (-34.8868, 9.1573) -> (-34.8868, 9.9883)
  line L505 (-32.8858, 9.0255) -> (-32.3868, 9.0255)
  line L506 (-32.3868, 9.0255) -> (-32.3868, 8.0745)
  line L507 (-32.3868, 8.0745) -> (-32.8858, 7.5731)
  line L508 (-32.8858, 7.5731) -> (-33.6368, 7.5731)
  line L509 (-33.6368, 7.5731) -> (-34.0205, 7.9568)
  line L510 (-34.0205, 7.9568) -> (-33.9687, 7.985)
  line L511 (-33.9687, 7.985) -> (-34.0699, 8.7666)
  line L512 (-34.0699, 8.7666) -> (-34.1358, 8.736)
  line L513 (-34.1358, 8.736) -> (-34.1358, 9.0255)
  line L514 (-34.1358, 9.0255) -> (-33.6532, 9.0255)
  line L515 (-33.6532, 9.0255) -> (-33.6532, 8.3993)
  line L516 (-33.6532, 8.3993) -> (-32.8858, 8.3993)
  line L517 (-32.8858, 8.3993) -> (-32.8858, 9.0255)
  line L518 (-34.8868, 7.4883) -> (-34.8868, 8.3782)
  line L519 (-34.8868, 8.3782) -> (-34.1358, 8.736)
  line L520 (-34.1358, 8.736) -> (-34.1358, 8.0745)
  line L521 (-34.1358, 8.0745) -> (-34.0205, 7.9568)
  line L522 (-34.0205, 7.9568) -> (-34.8868, 7.4883)
  line L523 (-34.3877, 6.3631) -> (-34.3877, 5.6475)
  line L524 (-34.3877, 5.6475) -> (-34.8868, 5.6475)
  line L525 (-34.8868, 5.6475) -> (-34.8868, 6.695)
  line L526 (-34.8868, 6.695) -> (-34.3877, 7.1941)
  line L527 (-34.3877, 7.1941) -> (-32.8858, 7.1941)
  line L528 (-32.8858, 7.1941) -> (-32.3868, 6.695)
  line L529 (-32.3868, 6.695) -> (-32.3868, 6.3631)
  line L530 (-32.3868, 6.3631) -> (-34.3877, 6.3631)
  line L531 (-33.5002, 5.9205) -> (-33.5002, 4.7788)
  line L532 (-33.5002, 4.7788) -> (-34.8868, 4.7788)
  line L533 (-34.8868, 4.7788) -> (-34.8868, 5.5156)
  line L534 (-34.8868, 5.5156) -> (-33.9969, 5.5156)
  line L535 (-33.9969, 5.5156) -> (-33.9969, 5.9205)
  line L536 (-33.9969, 5.9205) -> (-33.5002, 5.9205)
  line L537 (-32.8858, 6.2313) -> (-32.3868, 6.2313)
  line L538 (-32.3868, 6.2313) -> (-32.3868, 5.2143)
  line L539 (-32.3868, 5.2143) -> (-32.8858, 4.7788)
  line L540 (-32.8858, 4.7788) -> (-33.1353, 4.7788)
  line L541 (-33.1353, 4.7788) -> (-33.1353, 5.6098)
  line L542 (-33.1353, 5.6098) -> (-32.8858, 5.6098)
  line L543 (-32.8858, 5.6098) -> (-32.8858, 6.2313)
  line L544 (-39.9413, 32.5907) -> (-37.4413, 32.5907)
  line L545 (-37.4413, 32.5907) -> (-37.4413, 31.7597)
  line L546 (-37.4413, 31.7597) -> (-39.9413, 31.7597)
  line L547 (-39.9413, 31.7597) -> (-39.9413, 32.5907)
  line L548 (-37.9403, 31.6279) -> (-37.4413, 31.6279)
  line L549 (-37.4413, 31.6279) -> (-37.4413, 30.6769)
  line L550 (-37.4413, 30.6769) -> (-37.9403, 30.1755)
  line L551 (-37.9403, 30.1755) -> (-38.6913, 30.1755)
  line L552 (-38.6913, 30.1755) -> (-39.075, 30.5592)
  line L553 (-39.075, 30.5592) -> (-39.0232, 30.5874)
  line L554 (-39.0232, 30.5874) -> (-39.1244, 31.369)
  line L555 (-39.1244, 31.369) -> (-39.1903, 31.3384)
  line L556 (-39.1903, 31.3384) -> (-39.1903, 31.6279)
  line L557 (-39.1903, 31.6279) -> (-38.7077, 31.6279)
  line L558 (-38.7077, 31.6279) -> (-38.7077, 31.0017)
  line L559 (-38.7077, 31.0017) -> (-37.9403, 31.0017)
  line L560 (-37.9403, 31.0017) -> (-37.9403, 31.6279)
  line L561 (-39.9413, 30.0907) -> (-39.9413, 30.9806)
  line L562 (-39.9413, 30.9806) -> (-39.1903, 31.3384)
  line L563 (-39.1903, 31.3384) -> (-39.1903, 30.6769)
  line L564 (-39.1903, 30.6769) -> (-39.075, 30.5592)
  line L565 (-39.075, 30.5592) -> (-39.9413, 30.0907)
  line L566 (-37.9474, 28.2546) -> (-37.9474, 28.5724)
  line L567 (-37.9474, 28.5724) -> (-37.4413, 28.5724)
  line L568 (-37.4413, 28.5724) -> (-37.4413, 27.9274)
  line L569 (-37.4413, 27.9274) -> (-37.9403, 27.4212)
  line L570 (-37.9403, 27.4212) -> (-39.4493, 27.4212)
  line L571 (-39.4493, 27.4212) -> (-39.9413, 27.9274)
  line L572 (-39.9413, 27.9274) -> (-39.9413, 28.5724)
  line L573 (-39.9413, 28.5724) -> (-39.4328, 28.5724)
  line L574 (-39.4328, 28.5724) -> (-39.4328, 28.2546)
  line L575 (-39.4328, 28.2546) -> (-37.9474, 28.2546)
  line L576 (-39.4328, 29.0173) -> (-39.4328, 28.7042)
  line L577 (-39.4328, 28.7042) -> (-39.9413, 28.7042)
  line L578 (-39.9413, 28.7042) -> (-39.9413, 29.3445)
  line L579 (-39.9413, 29.3445) -> (-39.4493, 29.8506)
  line L580 (-39.4493, 29.8506) -> (-37.9403, 29.8506)
  line L581 (-37.9403, 29.8506) -> (-37.4413, 29.3445)
  line L582 (-37.4413, 29.3445) -> (-37.4413, 28.7042)
  line L583 (-37.4413, 28.7042) -> (-37.9474, 28.7042)
  line L584 (-37.9474, 28.7042) -> (-37.9474, 29.0173)
  line L585 (-37.9474, 29.0173) -> (-39.4328, 29.0173)
  line L586 (-37.9403, 25.458) -> (-37.9403, 26.0747)
  line L587 (-37.9403, 26.0747) -> (-37.4413, 26.0747)
  line L588 (-37.4413, 26.0747) -> (-37.4413, 25.1096)
  line L589 (-37.4413, 25.1096) -> (-37.9403, 24.6081)
  line L590 (-37.9403, 24.6081) -> (-38.4488, 24.6081)
  line L591 (-38.4488, 24.6081) -> (-38.6983, 24.8577)
  line L592 (-38.6983, 24.8577) -> (-38.9502, 24.6081)
  line L593 (-38.9502, 24.6081) -> (-39.4422, 24.6081)
  line L594 (-39.4422, 24.6081) -> (-39.9413, 25.1096)
  line L595 (-39.9413, 25.1096) -> (-39.9413, 26.0747)
  line L596 (-39.9413, 26.0747) -> (-39.4422, 26.0747)
  line L597 (-39.4422, 26.0747) -> (-39.4422, 25.458)
  line L598 (-39.4422, 25.458) -> (-38.9078, 25.458)
  line L599 (-38.9078, 25.458) -> (-38.9078, 26.0747)
  line L600 (-38.9078, 26.0747) -> (-38.4723, 26.0747)
  line L601 (-38.4723, 26.0747) -> (-38.4723, 25.458)
  line L602 (-38.4723, 25.458) -> (-37.9403, 25.458)
  line L603 (-37.4413, 27.0375) -> (-37.4413, 26.2065)
  line L604 (-37.4413, 26.2065) -> (-39.9413, 26.2065)
  line L605 (-39.9413, 26.2065) -> (-39.9413, 27.0375)
  line L606 (-39.9413, 27.0375) -> (-37.4413, 27.0375)
  line L607 (-37.9474, 22.6849) -> (-37.9474, 23.0027)
  line L608 (-37.9474, 23.0027) -> (-37.4413, 23.0027)
  line L609 (-37.4413, 23.0027) -> (-37.4413, 22.3577)
  line L610 (-37.4413, 22.3577) -> (-37.9403, 21.8516)
  line L611 (-37.9403, 21.8516) -> (-39.4493, 21.8516)
  line L612 (-39.4493, 21.8516) -> (-39.9413, 22.3577)
  line L613 (-39.9413, 22.3577) -> (-39.9413, 23.0027)
  line L614 (-39.9413, 23.0027) -> (-39.4328, 23.0027)
  line L615 (-39.4328, 23.0027) -> (-39.4328, 22.6849)
  line L616 (-39.4328, 22.6849) -> (-37.9474, 22.6849)
  line L617 (-39.4328, 23.4476) -> (-39.4328, 23.1345)
  line L618 (-39.4328, 23.1345) -> (-39.9413, 23.1345)
  line L619 (-39.9413, 23.1345) -> (-39.9413, 23.7748)
  line L620 (-39.9413, 23.7748) -> (-39.4493, 24.2809)
  line L621 (-39.4493, 24.2809) -> (-37.9403, 24.2809)
  line L622 (-37.9403, 24.2809) -> (-37.4413, 23.7748)
  line L623 (-37.4413, 23.7748) -> (-37.4413, 23.1345)
  line L624 (-37.4413, 23.1345) -> (-37.9474, 23.1345)
  line L625 (-37.9474, 23.1345) -> (-37.9474, 23.4476)
  line L626 (-37.9474, 23.4476) -> (-39.4328, 23.4476)
  line L627 (-38.1145, 20.9405) -> (-38.1145, 20.0742)
  line L628 (-38.1145, 20.0742) -> (-39.9413, 20.0742)
  line L629 (-39.9413, 20.0742) -> (-39.9413, 20.9405)
  line L630 (-39.9413, 20.9405) -> (-38.1145, 20.9405)
  line L631 (-37.4413, 21.5903) -> (-37.4413, 19.4222)
  line L632 (-37.4413, 19.4222) -> (-37.9851, 19.4222)
  line L633 (-37.9851, 19.4222) -> (-37.9851, 21.5903)
  line L634 (-37.9851, 21.5903) -> (-37.4413, 21.5903)
  line L635 (-39.4069, 19.1397) -> (-39.4069, 18.8902)
  line L636 (-39.4069, 18.8902) -> (-37.9733, 18.8902)
  line L637 (-37.9733, 18.8902) -> (-37.9733, 19.1397)
  line L638 (-37.9733, 19.1397) -> (-37.4413, 19.1397)
  line L639 (-37.4413, 19.1397) -> (-37.4413, 17.8073)
  line L640 (-37.4413, 17.8073) -> (-37.9733, 17.8073)
  line L641 (-37.9733, 17.8073) -> (-37.9733, 18.0592)
  line L642 (-37.9733, 18.0592) -> (-39.4069, 18.0592)
  line L643 (-39.4069, 18.0592) -> (-39.4069, 17.8073)
  line L644 (-39.4069, 17.8073) -> (-39.9413, 17.8073)
  line L645 (-39.9413, 17.8073) -> (-39.9413, 19.1397)
  line L646 (-39.9413, 19.1397) -> (-39.4069, 19.1397)
  line L647 (-39.9413, 16.6091) -> (-39.9413, 16.941)
  line L648 (-39.9413, 16.941) -> (-39.4422, 17.4401)
  line L649 (-39.4422, 17.4401) -> (-37.9403, 17.4401)
  line L650 (-37.9403, 17.4401) -> (-37.4413, 16.941)
  line L651 (-37.4413, 16.941) -> (-37.4413, 16.6091)
  line L652 (-37.4413, 16.6091) -> (-39.9413, 16.6091)
  line L653 (-37.9403, 16.4773) -> (-37.4413, 16.4773)
  line L654 (-37.4413, 16.4773) -> (-37.4413, 15.5898)
  line L655 (-37.4413, 15.5898) -> (-37.9403, 15.0907)
  line L656 (-37.9403, 15.0907) -> (-38.4441, 15.0907)
  line L657 (-38.4441, 15.0907) -> (-38.4441, 15.9241)
  line L658 (-38.4441, 15.9241) -> (-37.9403, 15.9241)
  line L659 (-37.9403, 15.9241) -> (-37.9403, 16.4773)
  line L660 (-39.9413, 16.4773) -> (-39.4422, 16.4773)
  line L661 (-39.4422, 16.4773) -> (-39.4422, 15.9241)
  line L662 (-39.4422, 15.9241) -> (-39.0773, 15.9241)
  line L663 (-39.0773, 15.9241) -> (-39.0773, 15.0907)
  line L664 (-39.0773, 15.0907) -> (-39.4422, 15.0907)
  line L665 (-39.4422, 15.0907) -> (-39.9413, 15.5898)
  line L666 (-39.9413, 15.5898) -> (-39.9413, 16.4773)
  line L667 (-39.9413, 13.1486) -> (-39.0044, 13.1486)
  line L668 (-39.0044, 13.1486) -> (-39.0044, 14.2291)
  line L669 (-39.0044, 14.2291) -> (-38.51, 14.7282)
  line L670 (-38.51, 14.7282) -> (-37.9403, 14.7282)
  line L671 (-37.9403, 14.7282) -> (-37.4413, 14.2291)
  line L672 (-37.4413, 14.2291) -> (-37.4413, 13.9467)
  line L673 (-37.4413, 13.9467) -> (-38.3287, 13.9467)
  line L674 (-38.3287, 13.9467) -> (-38.3287, 12.7979)
  line L675 (-38.3287, 12.7979) -> (-38.8325, 12.3129)
  line L676 (-38.8325, 12.3129) -> (-39.4422, 12.3129)
  line L677 (-39.4422, 12.3129) -> (-39.9413, 12.812)
  line L678 (-39.9413, 12.812) -> (-39.9413, 13.1486)
  line L679 (-39.1903, 14.7282) -> (-39.1903, 13.8972)
  line L680 (-39.1903, 13.8972) -> (-39.4893, 13.8972)
  line L681 (-39.4893, 13.8972) -> (-39.4893, 13.2805)
  line L682 (-39.4893, 13.2805) -> (-39.9413, 13.2805)
  line L683 (-39.9413, 13.2805) -> (-39.9413, 14.3092)
  line L684 (-39.9413, 14.3092) -> (-39.4422, 14.7282)
  line L685 (-39.4422, 14.7282) -> (-39.1903, 14.7282)
  line L686 (-37.8909, 13.8148) -> (-37.4413, 13.8148)
  line L687 (-37.4413, 13.8148) -> (-37.4413, 12.8144)
  line L688 (-37.4413, 12.8144) -> (-37.8768, 12.3812)
  line L689 (-37.8768, 12.3812) -> (-38.1404, 12.3812)
  line L690 (-38.1404, 12.3812) -> (-38.1404, 13.1486)
  line L691 (-38.1404, 13.1486) -> (-37.8909, 13.1486)
  line L692 (-37.8909, 13.1486) -> (-37.8909, 13.8148)
  point P0 (-38.3023, 0)
  constraints: 2 other
extrude "Extrusion10" cut sketch "Sketch3" against normal blind 0.2 contours L4 L5 L6 L7 L8 L9 L10 L11 | L12 L13 L14 L15 L16 L17 | L18 L19 L20 L21 | L22 L23 L24 L25 L26 L27 | L28 L29 L30 L31 L32 L33 L34 L35 | L36 L37 L38 L39 L40 L41 | L42 L43 L44 L45 L46 L47 | L48 L49 L50 L51 | L52 L53 L54 L55 | L56 L57 L58 L59 | L60 L61 L62 L63 L64 L65 L66 L67 L68 L69 L70 L71 | L72 L73 L74 L75 L76 L77 L78 L79 L80 L81 L82 L83 L84 L85 L86 L87 L88 | L89 L90 L91 L92 | L93 L94 L95 L96 | L97 L98 L99 L100 L101 L102 | L103 L104 L105 L106 L107 L108 L109 L110 | L111 L112 L113 L114 L115 L116 | L117 L118 L119 L120 L121 L122 | L123 L124 L125 L126 L127 L128 L129 L130 | L131 L132 L133 L134 L135 L136 | L137 L138 L139 L140 L141 L142 L143 L144 L145 L146 L147 L148 | L149 L150 L151 L152 | L153 L154 L155 L156 L157 L158 | L159 L160 L161 L162 L163 L164 L165 L166 | L167 L168 L169 L170 | L171 L172 L173 L174 L175 L176 | L177 L178 L179 L180 | L181 L182 L183 L184 | L185 L186 L187 L188 L189 L190 L191 L192 | L193 L194 L195 L196 L197 L198 | L199 L200 L201 L202 L203 L204 | L205 L206 L207 L208 | L209 L210 L211 L212 | L213 L214 L215 L216 | L217 L218 L219 L220 | L221 L222 L223 L224 | L225 L226 L227 L228 | L229 L230 L231 L232 | L233 L234 L235 L236 L237 L238 L239 L240 | L241 L242 L243 L244 | L245 L246 L247 L248 L249 L250 | L251 L252 L253 L254 | L255 L256 L257 L258 | L259 L260 L261 L262 L263 L264 L265 L266 | L267 L268 L269 L270 L271 L272 | L273 L274 L275 L276 L277 L278 | L279 L280 L281 L282 | L283 L284 L285 L286 L287 L288 L289 L290 L291 L292 L293 L294 L295 | L300 L296 L297 L298 L299 | L301 L302 L303 L304 L305 L306 L307 L308 L309 L310 L311 | L312 L313 L314 L315 L316 L317 L318 | L319 L320 L321 L322 | L323 L324 L325 L326 L327 L328 L329 L330 | L331 L332 L333 L334 L335 L336 L337 L338 | L339 L340 L341 L342 L343 L344 L345 L346 L347 L348 L349 | L350 L351 L352 L353 L354 L355 L356 | L357 L358 L359 L360 | L361 L362 L363 L364 L365 L366 L367 L368 L369 L370 L371 L372 L373 | L374 L375 L376 L377 L378 L379 L380 | L381 L382 L383 L384 L385 L386 L387 | L388 L389 L390 L391 | L392 L393 L394 L395 | L396 L397 L398 L399 L400 L401 L402 L403 L404 L405 L406 L407 | L408 L409 L410 L411 L412 L413 | L414 L415 L416 L417 L418 L419 L420 | L421 L422 L423 L424 L425 L426 L427 | L428 L429 L430 L431 | L432 L433 L434 L435 | L436 L437 L438 L439 | L440 L441 L442 L443 L444 L445 L446 L447 L448 L449 L450 L451 | L452 L453 L454 L455 L456 L457 L458 | L459 L460 L461 L462 L463 L464 L465 | L466 L467 L468 L469 L470 L471 L472 L473 L474 L475 L476 L477 L478 L479 L480 L481 L482 | L483 L484 L485 L486 | L487 L488 L489 L490 L491 L492 L493 | L494 L495 L496 L497 L498 L499 L500 | L501 L502 L503 L504 | L505 L506 L507 L508 L509 L510 L511 L512 L513 L514 L515 L516 L517 | L522 L518 L519 L520 L521 | L523 L524 L525 L526 L527 L528 L529 L530 | L531 L532 L533 L534 L535 L536 | L537 L538 L539 L540 L541 L542 L543 | L544 L545 L546 L547 | L548 L549 L550 L551 L552 L553 L554 L555 L556 L557 L558 L559 L560 | L565 L561 L562 L563 L564 | L566 L567 L568 L569 L570 L571 L572 L573 L574 L575 | L576 L577 L578 L579 L580 L581 L582 L583 L584 L585 | L586 L587 L588 L589 L590 L591 L592 L593 L594 L595 L596 L597 L598 L599 L600 L601 L602 | L603 L604 L605 L606 | L607 L608 L609 L610 L611 L612 L613 L614 L615 L616 | L617 L618 L619 L620 L621 L622 L623 L624 L625 L626 | L627 L628 L629 L630 | L631 L632 L633 L634 | L635 L636 L637 L638 L639 L640 L641 L642 L643 L644 L645 L646 | L647 L648 L649 L650 L651 L652 | L653 L654 L655 L656 L657 L658 L659 | L660 L661 L662 L663 L664 L665 L666 | L667 L668 L669 L670 L671 L672 L673 L674 L675 L676 L677 L678 | L679 L680 L681 L682 L683 L684 L685 | L686 L687 L688 L689 L690 L691 L692
body "Solid1"
